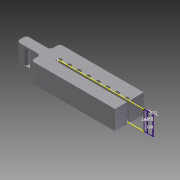
# Autodesk Inventor part: tensioners
Saved by Autodesk Inventor 2013 SP2 (Build 170200200, 200)
## iProperties
Created: 2015-11-30
Part Number: tensioners
Document SubType Name: Modeling
Designer: 2016ahoganso
Density: 1 g/cm^3
Material: Generic
Author: 2016ahoganso
Autodesk Inventor part; units mm, degrees
ref_plane "YZ Plane" through (0, 0, 0) normal (1, 0, 0) x (0, 1, 0)
ref_plane "XZ Plane" through (0, 0, 0) normal (0, 1, 0) x (-1, 0, 0)
ref_plane "XY Plane" through (0, 0, 0) normal (0, 0, 1) x (1, 0, 0)
sketch "Sketch1" plane through (0, 0, 0) normal (0, 0, 1) x (1, 0, 0)
  circle A0 centre (5.08, 17.272) radius 2.032
  arc A1 (11.1789, 13.4752) -> (0, 12.192) centre (5.08, 17.272) ccw
  line L0 (11.9198, 12.192) -> (38.8802, 12.192)
  circle A2 centre (45.72, 17.272) radius 2.032
  arc A3 (50.8, 12.192) -> (39.6211, 13.4752) centre (45.72, 17.272) ccw
  line L1 (0, 12.192) -> (0, 2.032)
  line L2 (50.8, 12.192) -> (50.8, 2.032)
  line L3 (11.9198, 12.192) -> (12.7, 12.192)
  line L4 (11.1789, 13.4752) -> (11.9198, 12.192)
  line L5 (38.8802, 12.192) -> (39.6211, 13.4752)
  line L6 (6.35, 2.032) -> (44.45, 2.032)
  circle A4 centre (0, -4.318) radius 2.032
  circle A5 centre (50.8, -4.318) radius 2.032
  arc A6 (0, 2.032) -> (6.0161, -6.35) centre (0, -4.318) ccw
  arc A7 (44.7839, -6.35) -> (50.8, 2.032) centre (50.8, -4.318) ccw
  line L7 (6.35, 2.032) -> (6.35, -6.096)
  line L8 (6.35, -6.096) -> (6.0161, -6.35)
  line L9 (44.45, 2.032) -> (44.2342, 2.032)
  line L10 (44.45, 2.032) -> (44.45, -6.096)
  line L11 (44.45, -6.096) -> (44.7839, -6.35)
  line L12 (11.9198, 12.192) -> (0, 12.192)
  line L13 (38.8802, 12.192) -> (50.8, 12.192)
  line L14 (50.8, 2.032) -> (44.45, 2.032)
  line L15 (6.35, 2.032) -> (0, 2.032)
  point P0 (10.16, 12.192)
  point P1 (10.16, 2.032)
  dimension "d28" = 11.9198
  dimension "d29" = 4.064
  dimension "d30" = 10.16
  dimension "d31" = 50.8
  dimension "d100" = 38.1
  constraints: 33 end point, 8 centre point, 8 point on circle, 4 coincident, 3 point on line, 2 perpendicular, 2 tangent, 1 collinear, 1 parallel, 2 other
  measures "d28" distance of L0.start L1.start
  measures "d29" diameter of A0
  measures "d30" distance between parallel lines of L0 L6
  measures "d31" distance between parallel lines of L2 L1
  measures "d100" distance of L6.start L6.end
extrude "Extrusion1" add sketch "Sketch1" along normal blind 6.35 contours L12 L0 L13 L2 L14 L6 L15 L1
sketch "Sketch2" plane through (0, 0, 6.35) normal (0, 0, 1) x (1, 0, 0)
  line L0 (0, 12.192) -> (50.8, 12.192) projected
  line L1 (50.8, 2.032) -> (0, 2.032) projected
  line L2 (0, 2.032) -> (50.8, 2.032)
  line L3 (50.8, 2.032) -> (50.8, 12.192)
  line L4 (50.8, 12.192) -> (0, 12.192)
  line L5 (0, 12.192) -> (0, 2.032)
  line L6 (0, 2.032) -> (2.54, 2.032)
  line L7 (2.54, 12.192) -> (0, 12.192)
  line L8 (0, 12.192) -> (0, 2.032)
  line L9 (2.54, 12.192) -> (5.08, 12.192)
  line L10 (5.08, 2.032) -> (2.54, 2.032)
  line L11 (5.08, 12.192) -> (7.62, 12.192)
  line L12 (7.62, 2.032) -> (5.08, 2.032)
  line L13 (7.62, 12.192) -> (10.16, 12.192)
  line L14 (10.16, 2.032) -> (7.62, 2.032)
  line L15 (10.16, 12.192) -> (12.7, 12.192)
  line L16 (12.7, 2.032) -> (10.16, 2.032)
  line L17 (12.7, 12.192) -> (15.24, 12.192)
  line L18 (15.24, 2.032) -> (12.7, 2.032)
  line L19 (15.2625, 12.192) -> (17.8025, 12.192)
  line L20 (17.8025, 2.032) -> (15.2625, 2.032)
  line L21 (17.8025, 12.192) -> (20.3425, 12.192)
  line L22 (20.3425, 2.032) -> (17.8025, 2.032)
  line L23 (20.3425, 12.192) -> (22.8825, 12.192)
  line L24 (22.8825, 2.032) -> (20.3425, 2.032)
  line L25 (22.8825, 12.192) -> (25.4225, 12.192)
  line L26 (25.4225, 2.032) -> (22.8825, 2.032)
  line L27 (25.4225, 12.192) -> (27.9625, 12.192)
  line L28 (27.9625, 2.032) -> (25.4225, 2.032)
  line L29 (27.9625, 12.192) -> (30.5025, 12.192)
  line L30 (30.5025, 2.032) -> (27.9625, 2.032)
  line L31 (30.5025, 12.192) -> (33.0425, 12.192)
  line L32 (33.0425, 2.032) -> (30.5025, 2.032)
  line L33 (33.0425, 12.192) -> (35.5825, 12.192)
  line L34 (35.5825, 2.032) -> (33.0425, 2.032)
  line L35 (35.5375, 12.192) -> (38.0775, 12.192)
  line L36 (38.0775, 2.032) -> (35.5375, 2.032)
  line L37 (38.0775, 12.192) -> (40.6175, 12.192)
  line L38 (40.6175, 2.032) -> (38.0775, 2.032)
  line L39 (40.6175, 12.192) -> (43.1575, 12.192)
  line L40 (43.1575, 2.032) -> (40.6175, 2.032)
  line L41 (43.1575, 12.192) -> (45.6975, 12.192)
  line L42 (45.6975, 2.032) -> (43.1575, 2.032)
  line L43 (45.6975, 12.192) -> (48.2375, 12.192)
  line L44 (48.2375, 2.032) -> (45.6975, 2.032)
  line L45 (48.2375, 12.192) -> (50.7775, 12.192)
  line L46 (50.7775, 2.032) -> (48.2375, 2.032)
  line L47 (33.0425, 12.192) -> (35.5825, 12.192)
  line L48 (35.5825, 2.032) -> (33.0425, 2.032)
  line L49 (50.7775, 12.192) -> (50.7775, 2.032)
  line L50 (48.2375, 12.192) -> (50.7775, 12.192)
  line L51 (50.7775, 2.032) -> (48.2375, 2.032)
  line L52 (50.7775, 2.032) -> (50.7775, 12.192)
  line L53 (50.7775, 2.032) -> (50.7775, 12.192)
  line L54 (45.6975, 12.192) -> (48.2375, 12.192)
  line L55 (48.2375, 2.032) -> (45.6975, 2.032)
  line L56 (43.1575, 12.192) -> (45.6975, 12.192)
  line L57 (45.6975, 2.032) -> (43.1575, 2.032)
  line L58 (40.6175, 12.192) -> (43.1575, 12.192)
  line L59 (43.1575, 2.032) -> (40.6175, 2.032)
  line L60 (38.0775, 12.192) -> (40.6175, 12.192)
  line L61 (40.6175, 2.032) -> (38.0775, 2.032)
  line L62 (35.5375, 12.192) -> (38.0775, 12.192)
  line L63 (38.0775, 2.032) -> (35.5375, 2.032)
  point P0 (6.096, 2.032)
  point P1 (44.704, 2.032)
  point P2 (0, 0)
  point P3 (44.45, 2.032)
  point P4 (6.35, 2.032)
  point P5 (3.175, 12.192)
  point P6 (47.625, 12.192)
  point P7 (47.625, 2.032)
  point P8 (3.175, 2.032)
  dimension "d43" = 50.8
  constraints: 126 end point, 29 parallel, 28 horizontal, 2 perpendicular, 2 point on line
  measures "d43" distance of L1.end L1.start
extrude "Extrusion2" add sketch "Sketch2" along normal blind 1.2446
sketch "Sketch3" plane through (0, 0, 7.5946) normal (0, 0, 1) x (1, 0, 0)
  line L0 (0, 2.032) -> (0, 12.192) projected
  line L1 (50.8, 2.032) -> (0, 2.032) projected
  line L2 (50.8, 12.192) -> (50.8, 2.032) projected
  line L3 (0, 12.192) -> (50.8, 12.192) projected
  line L4 (50.8, 12.192) -> (47.244, 12.192)
  line L5 (47.244, 12.192) -> (47.244, 2.032)
  line L6 (47.244, 2.032) -> (50.8, 2.032)
  line L7 (50.8, 2.032) -> (50.8, 12.192)
  line L8 (47.244, 12.192) -> (45.72, 12.192)
  line L9 (45.72, 12.192) -> (45.72, 2.032)
  line L10 (45.72, 2.032) -> (47.244, 2.032)
  line L11 (47.244, 2.032) -> (47.244, 12.192)
  line L12 (50.8, 12.192) -> (50.292, 12.192)
  line L13 (50.292, 12.192) -> (47.752, 12.192)
  line L14 (47.752, 12.192) -> (47.752, 2.032)
  line L15 (47.752, 2.032) -> (50.292, 2.032)
  line L16 (50.292, 2.032) -> (50.292, 12.192)
  point P0 (0, 0)
  dimension "d71" = 3.556
  dimension "d72" = 1.524
  dimension "d73" = 0.508
  dimension "d74" = 2.54
  constraints: 26 end point, 6 parallel, 4 point on line, 3 horizontal, 3 perpendicular
  measures "d71" distance between parallel lines of L5 L7
  measures "d72" distance between parallel lines of L9 L11
  measures "d73" distance of L2.start L12.end
  measures "d74" distance between parallel lines of L14 L16
sketch "Sketch5" plane through (6.096, 2.032, 0) normal (0, -1, 0) x (1, 0, 0)
  line L0 (44.704, 7.5946) -> (-6.096, 7.5946) projected
  line L1 (-6.096, 6.35) -> (-6.096, 7.5946) projected
  line L2 (44.704, 6.35) -> (-6.096, 6.35) projected
  line L3 (44.704, 6.35) -> (41.148, 6.35)
  line L4 (41.656, 7.5946) -> (41.148, 6.35)
  line L5 (41.148, 6.35) -> (39.624, 6.35)
  line L6 (39.624, 6.35) -> (39.116, 7.5946)
  line L7 (44.196, 7.5946) -> (41.656, 7.5946)
  line L8 (36.576, 7.5946) -> (36.068, 6.35)
  line L9 (36.068, 6.35) -> (34.544, 6.35)
  line L10 (34.544, 6.35) -> (34.036, 7.5946)
  line L11 (39.116, 7.5946) -> (36.576, 7.5946)
  line L12 (31.496, 7.5946) -> (30.988, 6.35)
  line L13 (30.988, 6.35) -> (29.464, 6.35)
  line L14 (29.464, 6.35) -> (28.956, 7.5946)
  line L15 (34.036, 7.5946) -> (31.496, 7.5946)
  line L16 (26.416, 7.5946) -> (25.908, 6.35)
  line L17 (25.908, 6.35) -> (24.384, 6.35)
  line L18 (24.384, 6.35) -> (23.876, 7.5946)
  line L19 (28.956, 7.5946) -> (26.416, 7.5946)
  line L20 (21.336, 7.5946) -> (20.828, 6.35)
  line L21 (20.828, 6.35) -> (19.304, 6.35)
  line L22 (19.304, 6.35) -> (18.796, 7.5946)
  line L23 (23.876, 7.5946) -> (21.336, 7.5946)
  line L24 (16.256, 7.5946) -> (15.748, 6.35)
  line L25 (15.748, 6.35) -> (14.224, 6.35)
  line L26 (14.224, 6.35) -> (13.716, 7.5946)
  line L27 (18.796, 7.5946) -> (16.256, 7.5946)
  line L28 (11.176, 7.5946) -> (10.668, 6.35)
  line L29 (10.668, 6.35) -> (9.144, 6.35)
  line L30 (9.144, 6.35) -> (8.636, 7.5946)
  line L31 (13.716, 7.5946) -> (11.176, 7.5946)
  line L32 (6.096, 7.5946) -> (5.588, 6.35)
  line L33 (5.588, 6.35) -> (4.064, 6.35)
  line L34 (4.064, 6.35) -> (3.556, 7.5946)
  line L35 (8.636, 7.5946) -> (6.096, 7.5946)
  line L36 (1.016, 7.5946) -> (0.508, 6.35)
  line L37 (0.508, 6.35) -> (-1.016, 6.35)
  line L38 (-1.016, 6.35) -> (-1.524, 7.5946)
  line L39 (3.556, 7.5946) -> (1.016, 7.5946)
  line L40 (-4.064, 7.5946) -> (-4.572, 6.35)
  line L41 (-4.572, 6.35) -> (-6.096, 6.35)
  line L42 (-1.524, 7.5946) -> (-4.064, 7.5946)
  line L43 (-6.096, 6.35) -> (-6.096, 7.5946)
  line L44 (-4.064, 7.5946) -> (-6.096, 7.5946)
  line L45 (-1.524, 7.5946) -> (1.016, 7.5946)
  line L46 (3.556, 7.5946) -> (6.3889, 7.5946)
  line L47 (8.636, 7.5946) -> (11.6007, 7.5946)
  line L48 (13.716, 7.5946) -> (41.656, 7.5946)
  line L49 (3.556, 7.5946) -> (6.096, 7.5946)
  line L50 (8.636, 7.5946) -> (11.176, 7.5946)
  line L51 (13.716, 7.5946) -> (16.256, 7.5946)
  line L52 (18.796, 7.5946) -> (21.336, 7.5946)
  line L53 (23.876, 7.5946) -> (26.416, 7.5946)
  line L54 (28.956, 7.5946) -> (31.496, 7.5946)
  line L55 (34.036, 7.5946) -> (36.576, 7.5946)
  line L56 (39.116, 7.5946) -> (41.656, 7.5946)
  point P0 (38.608, 6.35)
  point P1 (-6.096, 0)
  dimension "d78" = 3.556
  dimension "d80" = 1.524
  dimension "d82" = 1.524
  dimension "d83" = 1.524
  dimension "d84" = 1.524
  dimension "d85" = 1.524
  dimension "d86" = 1.524
  dimension "d87" = 1.524
  dimension "d88" = 1.524
  dimension "d89" = 1.524
  dimension "d90" = 1.524
  constraints: 108 end point, 12 collinear, 6 point on line, 1 perpendicular
  measures "d78" distance of L2.start L3.end
  measures "d80" distance of L3.end L5.end
  measures "d82" distance of L8.end L9.end
  measures "d83" distance of L12.end L13.end
  measures "d84" distance of L16.end L17.end
  measures "d85" distance of L20.end L21.end
  measures "d86" distance of L24.end L25.end
  measures "d87" distance of L28.end L29.end
  measures "d88" distance of L32.end L33.end
  measures "d89" distance of L36.end L37.end
  measures "d90" distance of L40.end L1.start
extrude "Extrusion4" cut sketch "Sketch5" against normal blind 25.4 contours L4 L2 L6 L0 | L8 L2 L10 L0 | L12 L2 L14 L0 | L16 L2 L18 L0 | L20 L2 L22 L0 | L24 L2 L26 L0 | L28 L2 L30 L0 | L2 L34 L0 L32 | L2 L38 L0 L36 | L2 L1 L0 L40
sketch "Sketch9" plane through (0, 2.032, 0) normal (-1, 0, 0) x (0, 0, 1)
  line L0 (6.35, 0) -> (6.35, 10.16) projected
  line L1 (0, 10.16) -> (6.35, 10.16) projected
  line L2 (0, 10.16) -> (0, 0) projected
  line L3 (0, 0) -> (6.35, 0) projected
  point P0 (0, -2.032)
extrude "Extrusion6" add sketch "Sketch9" along normal blind 6.35
sketch "Sketch10" plane through (1.524, 2.032, 6.35) normal (0, 0, 1) x (1, 0, 0)
  line L0 (49.276, 0) -> (-7.874, 0) projected
  line L1 (-7.874, 10.16) -> (-1.524, 10.16)
  line L2 (-1.524, 10.16) -> (-1.524, 0)
  line L3 (-1.524, 0) -> (-7.874, 0)
  line L4 (-7.874, 0) -> (-7.874, 10.16)
  point P0 (-1.524, -2.032)
  dimension "d104" = 6.35
  constraints: 8 end point, 2 parallel, 1 horizontal, 1 perpendicular, 1 point on line
  measures "d104" distance of L2.end L3.end
extrude "Extrusion7" add sketch "Sketch10" along normal blind 8.89
sketch "Sketch11" plane through (0, 2.032, 6.35) normal (1, 0, 0) x (0, 0, -1)
  line L0 (6.35, 0) -> (-8.89, 0) projected
  line L1 (-8.89, 10.16) -> (-2.54, 10.16)
  line L2 (-2.54, 10.16) -> (-2.54, 0)
  line L3 (-2.54, 0) -> (-8.89, 0)
  line L4 (-8.89, 0) -> (-8.89, 10.16)
  point P0 (6.35, -2.032)
  dimension "d107" = 6.35
  constraints: 8 end point, 2 parallel, 1 horizontal, 1 perpendicular, 1 point on line
  measures "d107" distance of L2.end L3.end
extrude "Extrusion8" add sketch "Sketch11" along normal blind 38.1
sketch "Sketch12" plane through (50.8, 2.032, 0) normal (0, -1, 0) x (1, 0, 0)
  line L0 (-10.16, 6.35) -> (-10.668, 7.5946) projected
  line L1 (-10.668, 7.5946) -> (-13.208, 7.5946) projected
  line L2 (0, 0) -> (-57.15, 0) projected
  line L3 (0, 0) -> (0, 7.5946) projected
  line L4 (0, 7.5946) -> (-3.048, 7.5946) projected
  line L5 (-3.048, 7.5946) -> (-3.556, 6.35) projected
  line L6 (-3.556, 6.35) -> (-5.08, 6.35) projected
  line L7 (-5.08, 6.35) -> (-5.588, 7.5946) projected
  line L8 (-5.588, 7.5946) -> (-8.128, 7.5946) projected
  line L9 (-8.128, 7.5946) -> (-8.636, 6.35) projected
  line L10 (-8.636, 6.35) -> (-10.16, 6.35) projected
  line L11 (-12.7, 7.5946) -> (-12.7, 0)
  line L12 (0, 0) -> (-57.15, 0) projected
  point P0 (-50.8, 0)
  constraints: 2 end point, 2 point on line, 1 perpendicular
extrude "Extrusion9" cut sketch "Sketch12" against normal blind 38.1
sketch "Sketch13" plane through (-6.35, 2.032, 0) normal (-1, 0, 0) x (0, 0, 1)
  line L0 (15.24, 10.16) -> (10.16, 10.16)
  line L1 (8.89, 10.16) -> (15.24, 10.16) projected
  line L2 (0, 10.16) -> (5.08, 10.16)
  line L3 (7.5946, 10.16) -> (0, 10.16) projected
  line L4 (0, 0) -> (7.5946, 0) projected
  line L5 (10.16, 10.16) -> (5.08, 10.16)
  line L6 (5.08, 10.16) -> (5.08, 0)
  line L7 (5.08, 0) -> (10.16, 0)
  line L8 (10.16, 0) -> (10.16, 10.16)
  point P0 (0, -2.032)
  dimension "d112" = 5.08
  dimension "d113" = 5.08
  constraints: 12 end point, 3 point on line, 2 parallel, 1 horizontal, 1 perpendicular
  measures "d112" distance of L0.start L0.end
  measures "d113" distance of L2.start L2.end
extrude "Extrusion10" add sketch "Sketch13" along normal blind 12.7
sketch "Sketch14" plane through (-6.35, 2.032, 5.08) normal (0, 0, -1) x (-1, 0, 0)
  line L0 (12.7, 10.16) -> (12.7, 0) projected
  line L1 (0, 10.16) -> (12.7, 10.16) projected
  line L2 (12.7, 5.08) -> (7.62, 5.08)
  line L3 (7.62, 5.08) -> (7.62, 9.017)
  line L4 (7.62, 5.08) -> (7.62, 1.143)
  line L5 (7.62, 1.143) -> (5.715, 1.143)
  line L6 (5.715, 1.143) -> (5.715, 9.017)
  line L7 (5.715, 9.017) -> (7.62, 9.017)
  point P0 (-6.35, -2.032)
  dimension "d116" = 5.08
  dimension "d117" = 3.937
  dimension "d118" = 3.937
  dimension "d119" = 1.905
  constraints: 12 end point, 3 perpendicular, 2 parallel, 1 collinear, 1 midpoint
  measures "d116" distance of L2.start L2.end
  measures "d117" distance of L2.end L3.end
  measures "d118" distance of L2.end L4.end
  measures "d119" distance of L4.end L5.end
extrude "Extrusion11" cut sketch "Sketch14" against normal blind 12.7
fillet "Fillet7" radius 1.5875 1 edges at (-13.97, 7.112, 5.08)
fillet "Fillet8" radius 1.5875 1 edges at (-13.97, 7.112, 10.16)
fillet "Fillet9" radius 1.5875 6 edges at (-19.05, 7.112, 10.16) (-19.05, 7.112, 5.08) (-6.35, 7.112, 0) (-6.35, 7.112, 15.24) (-6.35, 7.112, 5.08) (-6.35, 7.112, 10.16)
body "Solid1"
